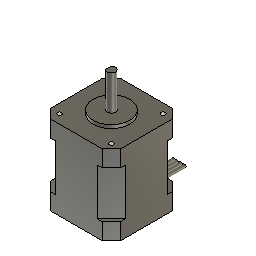
21to1 Reducer (Autodesk Fusion 360 archive; units mm, degrees)
design "NEMA 17 - 42 X 48 mm"
Autodesk Fusion 360 part; units mm, degrees
sketch "Sketch1" plane through (0, 0, 0) normal (0, 0, 1) x (1, 0, 0)
  line L0 (-21.15, 21.15) -> (21.15, 21.15)
  line L1 (21.15, 21.15) -> (21.15, -21.15)
  line L2 (21.15, -21.15) -> (-21.15, -21.15)
  line L3 (-21.15, -21.15) -> (-21.15, 21.15)
  line L4 (-21.15, -21.15) -> (21.15, 21.15)
  line L5 (21.15, 15.6) -> (21.15, -15.6)
  line L6 (15.6, 21.15) -> (-15.6, 21.15)
  line L7 (15.6, 21.15) -> (21.15, 15.6)
  line L8 (15.6, -21.15) -> (21.15, -15.6)
  line L9 (-15.6, 21.15) -> (-21.15, 15.6)
  line L10 (-15.6, -21.15) -> (-21.15, -15.6)
  dimension "d1" = 42.3
  dimension "d2" = 42.3
  dimension "d3" = 31.2
  dimension "d4" = 31.2
  constraint horizontal L0
  constraint vertical L1
  constraint horizontal L2
  constraint vertical L3
  constraint midpoint origin L4
  constraint perpendicular L0 L5
  constraint midpoint L1 L5
  constraint perpendicular L1 L6
  constraint midpoint L0 L6
  measures "d1" distance of L0.start L0.end
  measures "d2" distance of L0.start L2.end
  measures "d3" distance of L5.start L5.end
  measures "d4" distance of L6.start L6.end
extrude "Extrude1" add sketch "Sketch1" along normal blind 48 contours L0 L3 L4 L6 L7 L9 L10 | L1 L2 L4 L5 L7 L8 L10 makes body 1
sketch "Sketch2" plane through (0, 0, 48) normal (0, 0, 1) x (-1, 0, 0)
  line L0 (-15.6, 21.15) -> (-21.15, 15.6)
  line L1 (-21.15, 15.6) -> (-21.15, -15.6)
  line L2 (-21.15, -15.6) -> (-15.6, -21.15)
  line L3 (-15.6, -21.15) -> (15.6, -21.15)
  line L4 (15.6, -21.15) -> (21.15, -15.6)
  line L5 (21.15, -15.6) -> (21.15, 15.6)
  line L6 (21.15, 15.6) -> (15.6, 21.15)
  line L7 (15.6, 21.15) -> (-15.6, 21.15)
  line L8 (15.6, -15.6) -> (-15.6, -15.6)
  line L9 (-15.6, -15.6) -> (-15.6, 15.6)
  line L10 (-15.6, 15.6) -> (15.6, 15.6)
  line L11 (15.6, 15.6) -> (15.6, -15.6)
  line L12 (15.6, 15.6) -> (-15.6, -15.6)
  circle A0 centre (15.6, -15.6) radius 1.5
  circle A1 centre (-15.6, -15.6) radius 1.5
  circle A2 centre (15.6, 15.6) radius 1.5
  circle A3 centre (-15.6, 15.6) radius 1.5
  circle A4 centre (0, 0) radius 11.025
  circle A5 centre (0, 0) radius 2.5
  dimension "d7" = 31.2
  dimension "d8" = 31.2
  dimension "d9" = 3
  dimension "d12" = -31.2
  dimension "d13" = 31.2
  dimension "d16" = 22.05
  dimension "d19" = 5
  constraint horizontal L8
  constraint vertical L9
  constraint horizontal L10
  constraint vertical L11
  constraint midpoint A4.centre L12
  constraint coincident L8.start L11.end
  constraint coincident A4.centre A5.centre
  constraint concentric A4 A5
  measures "d7" distance of L8.start L8.end
  measures "d8" distance of L8.start L10.end
  measures "d9" diameter of A0
  measures "d16" diameter of A4
  measures "d19" diameter of A5
extrude "Extrude2" cut sketch "Sketch2" against normal blind 4.5 contours L8 L9 A1 | L8 L12 A1 | L9 L12 A1 | L8 L11 A0 | L8 L11 A0 | L9 L10 A3 | L9 L10 A3 | L11 L12 A2 | L10 L11 A2 | L10 L12 A2 bodies 1
extrude "Extrude3" add sketch "Sketch2" along normal blind 2 contours L12 A4 A5 | L12 A4 A5 | L12 A5 | L12 A5 bodies 1
extrude "Extrude4" add sketch "Sketch2" along normal blind 23 contours L12 A5 | L12 A5 bodies 1
sketch "Sketch3" plane through (0, 0, 71) normal (0, 0, 1) x (-1, 0, 0)
  circle A0 centre (0, 0) radius 2.5
  line L0 (-2.5, 0) -> (1.9, 0)
  line L1 (1.9, -1.6248) -> (1.9, 1.6248)
  circle A1 centre (0, 0) radius 2.5
  dimension "d22" = 4.4
  constraint coincident A0 L0.start
  constraint horizontal L0
  constraint coincident A0 L1.start
  constraint coincident A0 L1.end
  constraint perpendicular L0 L1
  constraint coincident A0.centre A1.centre
  constraint coincident L0.start A1
  measures "d22" distance of L0.start L0.end
extrude "Extrude5" cut sketch "Sketch3" against normal blind 15.25 contours A0 L1 A1 bodies 1
sketch "Sketch4" plane through (-18.375, -18.375, 0) normal (-0.707107, -0.707107, 0) x (0.707107, -0.707107, 0)
  line L0 (-3.9244, 0) -> (3.9244, 0)
  line L1 (3.9244, 0) -> (3.9244, 48)
  line L2 (3.9244, 48) -> (-3.9244, 48)
  line L3 (-3.9244, 48) -> (-3.9244, 0)
  line L4 (-3.9244, 10) -> (3.9244, 10)
  line L5 (-3.9244, 38) -> (3.9244, 38)
  line L6 (0, 48) -> (-22.0617, 48)
  line L7 (-6.25, 38) -> (6.25, 38)
  line L8 (6.25, 38) -> (6.25, 10)
  line L9 (6.25, 10) -> (-6.25, 10)
  line L10 (-6.25, 10) -> (-6.25, 38)
  dimension "d25" = 10
  dimension "d26" = 10
  dimension "d27" = 12.5
  dimension "d28" = 28
  constraint coincident L3 L4.start
  constraint coincident L1 L4.end
  constraint perpendicular L1 L4
  constraint coincident L3 L5.start
  constraint coincident L1 L5.end
  constraint perpendicular L1 L5
  constraint horizontal L7
  constraint vertical L8
  constraint horizontal L9
  constraint vertical L10
  constraint midpoint L5 L7
  measures "d25" distance of L0 L4
  measures "d26" distance of L5 L6
  measures "d27" distance of L7.start L7.end
  measures "d28" distance of L7.start L9.end
extrude "Extrude6" cut sketch "Sketch4" against normal blind 2 contours L3 L7 L9 L10 | L1 L3 L4 L5 L7 L9 | L1 L7 L8 L9 bodies 1
thread "Thread1" "ISO Metric profile 3.0 M3x0.5 6H" major diameter 3.086 minor diameter 2.529 pitch 0.5 angle 60 resizes the face on face at (-17.0925, -15.7494, 46.5) on face at (-17.0925, 15.7494, 45) on face at (14.1075, 15.7494, 45) on face at (14.1075, -15.4506, 45) on bodies 1
sketch "Sketch5" plane through (18.375, -18.375, 0) normal (0.707107, -0.707107, 0) x (0.707107, 0.707107, 0)
  line L0 (-3.9244, 0) -> (3.9244, 0)
  line L1 (3.9244, 0) -> (3.9244, 48)
  line L2 (3.9244, 48) -> (-3.9244, 48)
  line L3 (-3.9244, 48) -> (-3.9244, 0)
  line L4 (-6.2415, 38) -> (6.2585, 38)
  line L5 (6.2585, 38) -> (6.2585, 10)
  line L6 (6.2585, 10) -> (-6.2415, 10)
  line L7 (-6.2415, 10) -> (-6.2415, 38)
  line L8 (0, 48) -> (-22.0617, 48)
  line L9 (0, 48) -> (0.0085, 38)
  dimension "d33" = 12.5
  dimension "d34" = 28
  dimension "d35" = 10
  constraint horizontal L4
  constraint vertical L5
  constraint horizontal L6
  constraint vertical L7
  constraint coincident L8.start L9.start
  constraint midpoint L4 L9.end
  measures "d33" distance of L4.start L4.end
  measures "d34" distance of L4.start L6.end
  measures "d35" distance of L4 L8
extrude "Extrude7" cut sketch "Sketch5" against normal blind 2 contours L3 L4 L6 L7 | L1 L3 L4 L6 | L1 L4 L5 L6 bodies 1
sketch "Sketch6" plane through (18.375, 18.375, 0) normal (0.707107, 0.707107, 0) x (-0.707107, 0.707107, 0)
  line L0 (-3.9244, 0) -> (3.9244, 0)
  line L1 (3.9244, 0) -> (3.9244, 48)
  line L2 (3.9244, 48) -> (-3.9244, 48)
  line L3 (-3.9244, 48) -> (-3.9244, 0)
  line L4 (-6.25, 38) -> (6.25, 38)
  line L5 (6.25, 38) -> (6.25, 10)
  line L6 (6.25, 10) -> (-6.25, 10)
  line L7 (-6.25, 10) -> (-6.25, 38)
  line L8 (0, 38) -> (0, 48)
  dimension "d38" = 12.5
  dimension "d39" = 28
  dimension "d40" = 10
  constraint horizontal L4
  constraint vertical L5
  constraint horizontal L6
  constraint vertical L7
  constraint midpoint L4 L8.start
  constraint midpoint L2 L8.end
  constraint vertical L8
  measures "d38" distance of L4.start L4.end
  measures "d39" distance of L4.start L6.end
  measures "d40" distance of L8.start L8.end
extrude "Extrude8" cut sketch "Sketch6" against normal blind 2 contours L3 L4 L6 L7 | L1 L3 L4 L6 | L1 L4 L5 L6 bodies 1
sketch "Sketch7" plane through (-18.375, 18.375, 0) normal (-0.707107, 0.707107, 0) x (-0.707107, -0.707107, 0)
  line L0 (-3.9244, 0) -> (3.9244, 0)
  line L1 (3.9244, 0) -> (3.9244, 48)
  line L2 (3.9244, 48) -> (-3.9244, 48)
  line L3 (-3.9244, 48) -> (-3.9244, 0)
  line L4 (-6.25, 38) -> (6.25, 38)
  line L5 (6.25, 38) -> (6.25, 10)
  line L6 (6.25, 10) -> (-6.25, 10)
  line L7 (-6.25, 10) -> (-6.25, 38)
  line L8 (0, 48) -> (0, 38)
  dimension "d43" = 12.5
  dimension "d44" = 28
  dimension "d45" = 10
  constraint horizontal L4
  constraint vertical L5
  constraint horizontal L6
  constraint vertical L7
  constraint midpoint L2 L8.start
  constraint midpoint L4 L8.end
  constraint vertical L8
  measures "d43" distance of L4.start L4.end
  measures "d44" distance of L4.start L6.end
  measures "d45" distance of L8.start L8.end
extrude "Extrude9" cut sketch "Sketch7" against normal blind 2 contours L3 L4 L6 L7 | L1 L3 L4 L6 | L1 L4 L5 L6 bodies 1
sketch "Sketch8" plane through (0, 21.15, 0) normal (0, 1, 0) x (-1, 0, 0)
  line L0 (12.7716, 38) -> (15.6, 38)
  line L1 (15.6, 38) -> (15.6, 48)
  line L2 (15.6, 48) -> (-15.6, 48)
  line L3 (-15.6, 48) -> (-15.6, 38)
  line L4 (-15.6, 38) -> (-12.7716, 38)
  line L5 (-12.7716, 38) -> (-12.7716, 10)
  line L6 (-12.7716, 10) -> (-15.6, 10)
  line L7 (-15.6, 10) -> (-15.6, 0)
  line L8 (-15.6, 0) -> (15.6, 0)
  line L9 (15.6, 0) -> (15.6, 10)
  line L10 (15.6, 10) -> (12.7716, 10)
  line L11 (12.7716, 10) -> (12.7716, 38)
  circle A0 centre (-2.8917, 1.5852) radius 1
  circle A1 centre (-0.679, 1.5461) radius 1
  circle A2 centre (1.4517, 1.5004) radius 1
  circle A3 centre (3.6326, 1.655) radius 1
  dimension "d51" = 2
  dimension "d52" = 2
  dimension "d53" = 2
  dimension "d54" = 2
  measures "d51" diameter of A0
  measures "d52" diameter of A1
  measures "d53" diameter of A2
  measures "d54" diameter of A3
extrude "Extrude10" add sketch "Sketch8" along normal blind 20 separate body contours A0 | A1 | A2 | A3 makes body 2 at (1.893, 34.4833, 1.5353) makes body 3 at (-2.4505, 34.4833, 1.4505) makes body 4 at (-0.3197, 34.4833, 1.4962) makes body 5 at (-4.6313, 34.4833, 1.6051)

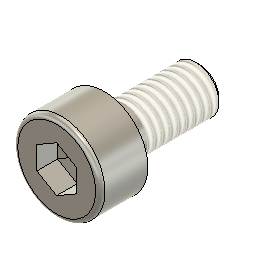
design "Hexagon Socket Head Cap Screw UNI EN ISO 4762 - M3 x 6 Steel 4.6 Plain"
description: Hexagon Socket Head Cap Screw UNI EN ISO 4762 - M3 x 6
part number: UNI EN ISO 4762 - M3 x 6 Steel 4.6 Plain
Autodesk Fusion 360 part; units mm, degrees
sketch "Sketch1" plane through (0, 0, 0) normal (0, 1, 0) x (1, 0, 0)
  line L0 (-1.5, 0) -> (-1.5, 6)
  line L1 (-1.5, 6) -> (0, 6)
  line L2 (0, 6) -> (0, -3)
  line L3 (-1.5, 0) -> (-2.75, 0)
  line L4 (-2.75, 0) -> (-2.75, -3)
  line L5 (-2.75, -3) -> (0, -3)
  dimension "d9" = 3
  dimension "d106" = 3
  dimension "d107" = 6
  dimension "d116" = 5.5
  constraint perpendicular L0 L1
  constraint collinear origin L1.end L2.end
  constraint perpendicular L0 L3
  constraint coincident origin L3
  constraint vertical L2
  constraint coincident L2 L5.end
  constraint perpendicular L2 L5
  measures "d106" distance of L3 L5
  measures "d107" distance of origin L1
revolve "Revolve1" add sketch "Sketch1" angle 360 about axis through (0, 0, -6) along (0, 0, 1)
ref_plane "WorkPlane1" through (0, 0, 3) normal (0, 0, 1) x (1, 0, 0)
sketch "Sketch6" plane through (0, 0, 3) normal (0, 0, 1) x (1, 0, 0)
  line L0 (-1.25, 0.7217) -> (-1.25, -0.7217)
  line L1 (-1.25, -0.7217) -> (0, -1.4434)
  line L2 (0, -1.4434) -> (1.25, -0.7217)
  line L3 (1.25, -0.7217) -> (1.25, 0.7217)
  line L4 (1.25, 0.7217) -> (0, 1.4434)
  line L5 (0, 1.4434) -> (-1.25, 0.7217)
  dimension "d117" = 2.5
  constraint vertical L0
  measures "d117" distance of L0 L3
extrude "Extrude1" cut sketch "Sketch6" against normal blind 1.3
extrude "Extrude2" cut 1 faces at (-0.4167, 0.2406, 1.7) along direction (0, 0, -1) blind 1.3 draft -85
fillet "Fillet4" radius 0.3 1 edges at (-2.5639, 0.9944, 3)
thread "Thread3" "ISO Metric profile 3.0 M3x0.5 M3x0.5 6g" major diameter 2.927 minor diameter 2.3555 pitch 0.5 angle 60 resizes the face on face at (-1.4925, 0.1494, -4) from (0, 0, -1.25) to (0, 0, -6)
sketch "Sketch7" plane through (0, 0, 0) normal (0, 1, 0) x (1, 0, 0)
  line L0 (-1.53, 6) -> (-1.53, 5.7)
  line L1 (-1.53, 5.7) -> (-1.23, 6)
  line L2 (0, 6) -> (0, -3)
  line L3 (-1.53, 6) -> (0, 6)
  dimension "d101" = 45
  dimension "d112" = 0.3
  dimension "d113" = 1.53
  constraint coincident L2.start L3.end
  constraint perpendicular L2 L3
  constraint coincident L1.end L3
  constraint perpendicular L0 L3
  measures "d101" angle of L0 L1
  measures "d112" distance of L0.end L3
  measures "d113" distance of L0 L2.start
revolve "Revolve3" cut sketch "Sketch7" angle 360 about axis through (0, 0, 1.75) along (0, 0, 1)
equation "d9 = adsk_nomdia"
equation "adsk_nomlen = 6.00 mm"
equation "adsk_headh = 3.00 mm"
equation "adsk_headdia = 5.50 mm"
equation "adsk_nomdia = 3.00 mm"
equation "adsk_philwidth = 2.50 mm"
equation "d31 = -adsk_phildepth"
equation "adsk_phildepth = 1.30 mm"
equation "d71 = adsk_headh"
equation "d76 = -adsk_phildepth"
equation "adsk_thrlen = 4.75 mm"
equation "d86 = adsk_nomdia * 0.1"
equation "adsk_startang = 45.00 deg"
equation "d101 = adsk_startang"
equation "adsk_pitch1 = 0.50 mm"
equation "adsk_startlen = 0.30 mm"
equation "d106 = adsk_headh"
equation "d107 = adsk_nomlen"
equation "d112 = adsk_startlen"
equation "d113 = adsk_nomdia * 0.51"
equation "d115 = min(adsk_thrlen; adsk_nomlen - 0.001 mm)"
equation "d116 = adsk_headdia"
equation "d117 = adsk_philwidth"
